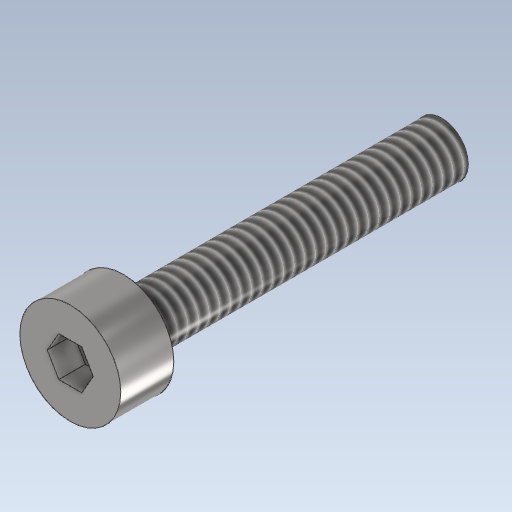
# Autodesk Inventor part: CSH-STH-M2-12
Saved by Autodesk Inventor 2020 (Build 240168000, 168)
## iProperties
Part Number: CSH-STH-M2-12
Material: チタン
Document SubType Name: Modeling
Designer: Masato Kubotera
Density: 5.93844 g/cm^3
Appearance: 半つや出し
Mass: 0.347 g
Surface Area: 1.27153 cm^2
Volume: 0.0584329 cm^3
Description: ReadyMade
Catalog Web Link: https://jp.misumi-ec.com/vona2/detail/221303734904/?HissuCode=CSH-STH-M2-12
Author: Masato Kubotera
Comments: Width across flats : 1.5
Autodesk Inventor part; units mm, degrees
ref_plane "YZ Plane" through (0, 0, 0) normal (1, 0, 0) x (0, 1, 0)
ref_plane "XZ Plane" through (0, 0, 0) normal (0, 1, 0) x (-1, 0, 0)
ref_plane "XY Plane" through (0, 0, 0) normal (0, 0, 1) x (1, 0, 0)
sketch "スケッチ1" plane through (0, 0, 0) normal (1, 0, 0) x (0, 1, 0)
  line L0 (0, 14) -> (0, 0)
  line L1 (0, 0) -> (1.9, 0)
  line L2 (1.9, 0) -> (1.9, 2)
  line L3 (1.9, 2) -> (1, 2)
  line L4 (1, 2) -> (1, 14)
  line L5 (1, 14) -> (0, 14)
  dimension "d2" = 2
  dimension "d10" = 12
  dimension "d11" = 2
  dimension "d12" = 3.8
  constraints: 12 end point, 5 perpendicular, 1 vertical
  measures "d2" distance of L1.end L2.end
  measures "d10" distance of L3.end L4.end
  measures "d11" diameter of L4 L0
  measures "d12" diameter of L2 L0
revolve "回転1" add sketch "スケッチ1" angle 360 about axis through (0, 0, 14) along (0, 0, -1)
thread "ねじ1" size "M2x0.4" class "6g" standard "ANSI Metric M Profile" full length
sketch "スケッチ2" plane through (0, 0, 0) normal (0, 0, -1) x (-1, 0, 0)
  line L0 (0, 0.866) -> (0.75, 0.433)
  line L1 (0.75, 0.433) -> (0.75, -0.433)
  line L2 (0.75, -0.433) -> (0, -0.866)
  line L3 (0, -0.866) -> (-0.75, -0.433)
  line L4 (-0.75, -0.433) -> (-0.75, 0.433)
  line L5 (-0.75, 0.433) -> (0, 0.866)
  circle A0 centre (0, 0) radius 1.9 projected
  line L6 (0, 1.9) -> (0, -1.9) construction
  dimension "d7" = 1.5
  constraints: 14 end point, 2 point on circle, 1 coincident, 1 midpoint, 1 point on line, 1 vertical, 13 other
  measures "d7" distance between parallel lines of L1 L4
extrude "押し出し1" cut sketch "スケッチ2" against normal blind 1 contours L0 L1 L2 L3 L4 L5
